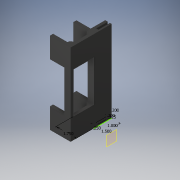
# Autodesk Inventor part: Suspension mount 2.0
Saved by Autodesk Inventor 2018.2 (Build 222227000, 227)
## iProperties
Created: 2018-02-01
Part Number: Suspension mount 2.0
Material: Acetal Resin, Black
Document SubType Name: Modeling
Designer: MIABo
Density: 1.425 g/cm^3
Appearance: Smooth - Black
Author: MIABo
Autodesk Inventor part; units mm, degrees
ref_plane "YZ Plane" through (0, 0, 0) normal (1, 0, 0) x (0, 1, 0)
ref_plane "XZ Plane" through (0, 0, 0) normal (0, 1, 0) x (-1, 0, 0)
ref_plane "XY Plane" through (0, 0, 0) normal (0, 0, 1) x (1, 0, 0)
sketch "Sketch1" plane through (0, 0, 0) normal (0, 1, 0) x (-1, 0, 0)
  line L0 (-51.9733, 36.6301) -> (-51.9733, 68.3801)
  line L1 (-65.3083, 74.7301) -> (-65.3083, 36.6301)
  line L2 (-65.3083, 36.6301) -> (-62.1333, 36.6301)
  line L3 (-62.1333, 36.6301) -> (-62.1333, 62.0301)
  line L4 (-62.1333, 62.0301) -> (-57.0533, 62.0301)
  line L5 (-57.0533, 62.0301) -> (-57.0533, 36.6301)
  line L6 (-57.0533, 36.6301) -> (-51.9733, 36.6301)
  line L7 (-51.9733, 68.3801) -> (-20.8583, 68.3801)
  line L8 (-20.8583, 68.3801) -> (-20.8583, 74.7301)
  line L9 (-20.8583, 74.7301) -> (-65.3083, 74.7301)
  dimension "d2" = 5.08
  dimension "d4" = 25.4
  dimension "d18" = 6.35
  dimension "d19" = 38.1
  dimension "d20" = 3.175
  dimension "d79" = 5.08
  dimension "d80" = 44.45
  constraints: 20 end point, 7 perpendicular, 1 horizontal, 1 parallel, 1 point on line, 1 vertical
  measures "d2" distance of L3.end L4.end
  measures "d4" distance of L2.end L3.end
  measures "d18" distance between parallel lines of L9 L7
  measures "d19" distance of L1.start L1.end
  measures "d20" distance of L1.end L2.end
  measures "d79" distance of L5.end L0.start
  measures "d80" distance of L8.end L1.start
extrude "Extrusion1" add sketch "Sketch1" along normal blind 177.8
ref_plane "Work Plane2" through (65.3083, -38.1, 36.6301) normal (1, 0, 0) x (0, 0, -1)
sketch "Sketch13" plane through (20.8583, 0, 74.7301) normal (0, 0, 1) x (1, 0, 0)
  line L0 (38.1, 0) -> (44.45, 0)
  line L1 (44.45, 0) -> (44.45, 177.8)
  line L2 (44.45, 177.8) -> (38.1, 177.8)
  line L3 (38.1, 177.8) -> (38.1, 0)
  line L4 (44.45, 0) -> (44.45, 177.8) projected
  line L5 (0, 177.8) -> (44.45, 177.8) projected
  line L6 (0, 0) -> (44.45, 0) projected
  point P0 (-20.8583, 0)
  point P1 (36.195, 177.8)
  point P2 (41.275, 177.8)
  point P3 (36.195, 0)
  point P4 (41.275, 0)
  point P5 (31.115, 0)
  dimension "d81" = 6.35
  constraints: 8 end point, 3 collinear, 2 parallel, 1 horizontal, 1 perpendicular
  measures "d81" distance between parallel lines of L1 L3
extrude "Extrusion2" add sketch "Sketch13" along normal blind 50.8
sketch "Sketch21" plane through (58.9583, 0, 74.7301) normal (-1, 0, 0) x (0, 0, 1)
  line L0 (50.8, 177.8) -> (50.8, 0) projected
  line L1 (50.8, 0) -> (44.45, 0)
  line L2 (44.45, 0) -> (44.45, 177.8)
  line L3 (44.45, 177.8) -> (50.8, 177.8)
  line L4 (50.8, 177.8) -> (50.8, 0)
  line L5 (0, 177.8) -> (50.8, 177.8) projected
  point P0 (-74.7301, 0)
  dimension "d91" = 6.35
  constraints: 8 end point, 2 parallel, 1 collinear, 1 horizontal, 1 perpendicular
  measures "d91" distance of L2.end L3.end
extrude "Extrusion10" add sketch "Sketch21" along normal blind 38.1
sketch "Sketch22" plane through (51.9733, 0, 68.3801) normal (0, 0, -1) x (-1, 0, 0)
  line L0 (31.115, 0) -> (31.115, 177.8) projected
  line L1 (0, 44.45) -> (31.115, 44.45)
  line L2 (31.115, 44.45) -> (31.115, 133.35)
  line L3 (31.115, 133.35) -> (0, 133.35)
  line L4 (0, 133.35) -> (0, 44.45)
  line L5 (0, 0) -> (31.115, 0) projected
  line L6 (0, 177.8) -> (31.115, 177.8) projected
  line L7 (0, 0) -> (0, 177.8) projected
  point P0 (51.9733, 0)
  dimension "d94" = 44.45
  dimension "d95" = 44.45
  constraints: 8 end point, 2 parallel, 1 collinear, 1 horizontal, 1 perpendicular, 1 point on line
  measures "d94" distance between parallel lines of L5 L1
  measures "d95" distance between parallel lines of L6 L3
extrude "Extrusion11" cut sketch "Sketch22" against normal blind 76.2 contours L1 L4 L3 L0
sketch "Sketch23" plane through (20.8583, 0, 74.7301) normal (0, 0, 1) x (1, 0, 0)
  line L0 (0, 177.8) -> (38.1, 177.8) projected
  line L1 (38.1, 177.8) -> (31.115, 177.8)
  line L2 (31.115, 177.8) -> (31.115, 0)
  line L3 (31.115, 0) -> (38.1, 0)
  line L4 (38.1, 0) -> (38.1, 177.8)
  line L5 (31.115, 133.35) -> (31.115, 44.45) projected
  line L6 (38.1, 0) -> (38.1, 177.8) projected
  line L7 (0, 0) -> (38.1, 0) projected
  point P0 (-20.8583, 0)
  constraints: 8 end point, 3 collinear, 2 parallel, 1 horizontal, 1 perpendicular
revolve "Revolution8" add sketch "Sketch23" angle 90 about axis through (58.9583, 0, 74.7301) along (0, 1, 0)
sketch "Sketch24" plane through (58.9583, 0, 119.1801) normal (0, 0, -1) x (-1, 0, 0)
  line L0 (0, 0) -> (0, 177.8) projected
  line L1 (0, 177.8) -> (38.1, 177.8) projected
  line L2 (0, 0) -> (6.985, 0)
  line L3 (6.985, 0) -> (6.985, 177.8)
  line L4 (6.985, 177.8) -> (0, 177.8)
  line L5 (0, 177.8) -> (0, 0)
  line L6 (6.985, 44.45) -> (6.985, 133.35) projected
  point P0 (58.9583, 0)
  constraints: 8 end point, 2 parallel, 1 collinear, 1 horizontal, 1 perpendicular, 1 point on line
revolve "Revolution9" add sketch "Sketch24" angle 90 about axis through (58.9583, 177.8, 119.1801) along (0, -1, 0)
sketch "Sketch25" plane through (65.3083, 0, 36.6301) normal (1, 0, 0) x (0, 0, -1)
  line L0 (-38.1, 44.45) -> (-82.55, 44.45)
  line L1 (-82.55, 44.45) -> (-82.55, 133.35)
  line L2 (-82.55, 133.35) -> (-38.1, 133.35)
  line L3 (-38.1, 133.35) -> (-38.1, 44.45)
  line L4 (-88.9, 0) -> (-88.9, 177.8) projected
  line L5 (-38.1, 133.35) -> (-38.1, 44.45) projected
  line L6 (0, 0) -> (-88.9, 0) projected
  line L7 (0, 177.8) -> (-88.9, 177.8) projected
  line L8 (-82.55, 44.45) -> (-82.55, 0) projected
  point P0 (36.6301, 0)
  dimension "d100" = 44.45
  dimension "d101" = 44.45
  constraints: 8 end point, 2 collinear, 2 parallel, 1 horizontal, 1 perpendicular
  measures "d100" distance between parallel lines of L6 L0
  measures "d101" distance between parallel lines of L7 L2
extrude "Extrusion12" cut sketch "Sketch25" against normal blind 76.2
body "Solid1"
